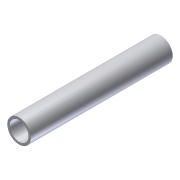
# Autodesk Inventor part: Conveyor_Roller_PVCPipe_size1.5
Saved by Autodesk Inventor 2012 (Build 160160000, 160)
## iProperties
Created: 2012-01-09
Part Number: Conveyor_Roller_PVCPipe_size1.5
Material: PVC-Piping
Document SubType Name: Modeling
Designer: JesseK
Mass: 316.881 g
Surface Area: 888.497 cm^2
Volume: 226.344 cm^3
Density: 1.4 g/cm^3
Author: JesseK
Autodesk Inventor part; units mm, degrees
ref_plane "YZ Plane" through (0, 0, 0) normal (1, 0, 0) x (0, 1, 0)
ref_plane "XZ Plane" through (0, 0, 0) normal (0, 1, 0) x (-1, 0, 0)
ref_plane "XY Plane" through (0, 0, 0) normal (0, 0, 1) x (1, 0, 0)
sketch "Sketch1" plane through (0, 0, 0) normal (0, 0, 1) x (1, 0, 0)
  circle A0 centre (0, 0) radius 25.4
  circle A1 centre (0, 0) radius 20.2184
  dimension "d0" = 50.8
  dimension "d2" = 40.4368
  constraints: 2 centre point, 2 coincident
  measures "d0" diameter of A0
  measures "d2" diameter of A1
extrude "Extrusion1" add sketch "Sketch1" along normal blind 304.8
body "Solid1"
